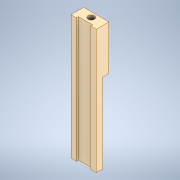
# Autodesk Inventor part: 5211_Bias_TxRx_Relative_Dovetail_Female_MPSv2_v4
Saved by Autodesk Inventor 2021 (Build 250183000, 183)
## iProperties
Created: 2020-11-13
Part Number: 5211_Bias_TxRx_Relative_Dovetail_Female_MPSv2_v4
Material: Polyethylene, High Density
Document SubType Name: Modeling
Designer: Admin
Density: 0.952 g/cm^3
Appearance: Smooth - Off-White
Author: Admin
Autodesk Inventor part; units mm, degrees
ref_plane "YZ Plane" through (0, 0, 0) normal (1, 0, 0) x (0, 1, 0)
ref_plane "XZ Plane" through (0, 0, 0) normal (0, 1, 0) x (-1, 0, 0)
ref_plane "XY Plane" through (0, 0, 0) normal (0, 0, 1) x (1, 0, 0)
sketch "Sketch1" plane through (0, 0, 0) normal (0, 0, 1) x (1, 0, 0)
  line L0 (0, 0) -> (47, 0)
  line L1 (47, 0) -> (47, -300)
  line L2 (47, -300) -> (0, -300)
  line L3 (0, -300) -> (0, 0)
  dimension "d0" = 47
  dimension "d1" = 300
  constraints: 8 end point, 2 parallel, 1 horizontal, 1 perpendicular
  measures "d0" distance of L1.end L2.end
  measures "d1" distance of L0.end L1.end
extrude "Extrusion1" add sketch "Sketch1" along normal blind 25.4
sketch "Sketch2" plane through (0, -300, 0) normal (0, -1, 0) x (1, 0, 0)
  line L0 (0, 0) -> (0, 25.4) projected
  line L1 (0, 25.4) -> (47, 25.4) projected
  line L2 (0, 0) -> (10, 0)
  line L3 (10, 0) -> (10, 21.4)
  line L4 (10, 25.4) -> (0, 25.4)
  line L5 (0, 25.4) -> (0, 0)
  line L6 (0, 0) -> (47, 0) projected
  line L7 (47, 0) -> (37, 0)
  line L8 (37, 0) -> (37, 25.4)
  line L9 (37, 25.4) -> (47, 25.4)
  line L10 (47, 25.4) -> (47, 0)
  line L11 (10, 25.4) -> (3.1941, 0)
  line L12 (10, 25.4) -> (36.296, 25.4) construction
  line L13 (37, 25.4) -> (43.8059, 0)
  line L14 (37, 25.4) -> (63.296, 25.4) construction
  line L15 (37, 25.4) -> (37, 21.4)
  line L16 (37, 21.4) -> (8.9282, 21.4)
  line L17 (37, 21.4) -> (38.0718, 21.4)
  line L18 (10, 25.4) -> (37, 25.4)
  dimension "d4" = 10
  dimension "d5" = 10
  dimension "d6" = 105
  dimension "d7" = 75
  dimension "d8" = 4
  constraints: 32 end point, 9 point on line, 5 horizontal, 4 parallel, 2 equal length, 2 perpendicular, 1 collinear
  measures "d4" distance of L4.end L4.start
  measures "d5" distance of L8.end L9.end
  measures "d6" angle of L11 L12
  measures "d7" angle of L13 L14
  measures "d8" distance of L8.end L15.end
extrude "Extrusion2" cut sketch "Sketch2" against normal blind 300 contours L1 L8 L16 L11 | L13 L17 L8
sketch "Sketch3" plane through (0, 0, 0) normal (0, 0, -1) x (-1, 0, 0)
  line L0 (-50.8, -30) -> (0, -30)
  line L1 (0, -30) -> (-50.8, -30)
  line L2 (0, 8.1) -> (0, -30)
  line L3 (-47, -30) -> (0, -30)
  line L4 (0, -15) -> (0, -30)
  line L5 (0, -30) -> (-47, -30)
  line L6 (-47, -30) -> (-47, -15)
  line L7 (-47, -15) -> (0, -15)
  line L8 (0, -15) -> (-47, -30) construction
  line L9 (0, -30) -> (-47, -15) construction
  line L10 (-47, 0) -> (0, 0)
  line L11 (0, 0) -> (-47, -15) construction
  line L12 (0, -15) -> (-47, 0) construction
  line L13 (-47, -15) -> (0, -15)
  line L14 (0, -15) -> (-47, -15)
  line L15 (0, 0) -> (0, -15)
  line L16 (-47, -15) -> (-47, 0)
  line L17 (-8.5, -22.5) -> (-8.5, -7.5)
  circle A0 centre (-8.5, -22.5) radius 1.5875
  circle A1 centre (-38.5, -22.5) radius 1.5875
  circle A2 centre (-38.5, -7.5) radius 1.5875
  circle A3 centre (-8.5, -7.5) radius 1.5875
  line L18 (-47, 0) -> (0, 0) projected
  line L19 (0, 0) -> (0, -122.988)
  line L20 (0, 0) -> (0, -300) projected
  line L21 (-50.8, -122.988) -> (0, -122.988)
  line L22 (0, -122.988) -> (-50.8, -122.988)
  line L23 (-47, -122.988) -> (0, -122.988)
  line L24 (0, -107.988) -> (0, -122.988)
  line L25 (0, -122.988) -> (-47, -122.988)
  line L26 (-47, -122.988) -> (-47, -107.988)
  line L27 (-47, -107.988) -> (0, -107.988)
  line L28 (0, -107.988) -> (-47, -122.988) construction
  line L29 (0, -122.988) -> (-47, -107.988) construction
  line L30 (-47, -92.988) -> (0, -92.988)
  line L31 (0, -92.988) -> (-47, -107.988) construction
  line L32 (0, -107.988) -> (-47, -92.988) construction
  line L33 (-47, -107.988) -> (0, -107.988)
  line L34 (0, -107.988) -> (-47, -107.988)
  line L35 (0, -92.988) -> (0, -107.988)
  line L36 (-47, -107.988) -> (-47, -92.988)
  line L37 (-8.5, -115.488) -> (-8.5, -100.488)
  circle A4 centre (-8.5, -115.488) radius 1.5875
  circle A5 centre (-38.5, -115.488) radius 1.5875
  circle A6 centre (-38.5, -100.488) radius 1.5875
  circle A7 centre (-8.5, -100.488) radius 1.5875
  line L38 (-16, -115.488) -> (-13.5, -115.488)
  line L39 (-13.5, -115.488) -> (-8.5, -115.488)
  line L40 (-31, -115.488) -> (-33.5, -115.488)
  line L41 (-33.5, -115.488) -> (-41, -115.488)
  line L42 (-41, -115.488) -> (-38.5, -115.488)
  point P0 (0, -6.35)
  point P1 (0, -30)
  point P2 (-27, -15)
  point P3 (-12, -15)
  point P4 (0, -15)
  point P5 (-10, 0)
  point P6 (0, -99.338)
  point P7 (-27, -107.988)
  point P8 (-12, -107.988)
  point P9 (0, -107.988)
  dimension "d11" = 15
  dimension "d12" = 15
  dimension "d13" = 3.175
  dimension "d14" = 3.175
  dimension "d15" = 3.175
  dimension "d16" = 3.175
  dimension "d17" = 122.988
  dimension "d18" = 15
  dimension "d19" = 15
  dimension "d20" = 3.175
  dimension "d21" = 3.175
  dimension "d22" = 3.175
  dimension "d23" = 3.175
  dimension "d30" = 5
  dimension "d31" = 7.5
  dimension "d32" = 2.5
  constraints: 82 end point, 8 centre point, 8 parallel, 4 coincident, 4 horizontal, 4 perpendicular, 3 point on line, 2 other
  measures "d11" distance of L3.start L6.end
  measures "d12" distance of L11.end L10.start
  measures "d13" diameter of A0
  measures "d14" diameter of A1
  measures "d15" diameter of A2
  measures "d16" diameter of A3
  measures "d17" distance of L18.end L19.end
  measures "d18" distance of L28.end L27.start
  measures "d19" distance of L33.start L32.end
  measures "d20" diameter of A4
  measures "d21" diameter of A5
  measures "d22" diameter of A6
  measures "d23" diameter of A7
  measures "d30" distance of L38.end L39.end
  measures "d31" distance of L40.end L41.end
  measures "d32" distance of L41.end L42.end
extrude "Extrusion3" cut sketch "Sketch3" against normal blind 10 contours A0 | A7 | A3 | A4 L39 L37 | L37 L39 A4 | A1 | A2 | L41 A5 | A5 L41 | A6
sketch "Sketch4" plane through (0, -300, 0) normal (0, -1, 0) x (1, 0, 0)
  line L0 (0, 0) -> (47, 0) projected
  line L1 (47, 0) -> (47, 25.4) projected
  line L2 (0, 0) -> (47, 0)
  line L3 (47, 0) -> (47, 12.7)
  line L4 (47, 12.7) -> (0, 12.7)
  line L5 (0, 12.7) -> (0, 0)
  dimension "d27" = 12.7
  constraints: 8 end point, 2 parallel, 1 horizontal, 1 midpoint, 1 perpendicular
  measures "d27" distance of L3.end L2.end
extrude "Extrusion4" cut sketch "Sketch4" against normal blind 160
sketch "Sketch7" plane through (0, 0, 0) normal (0, 1, 0) x (1, 0, 0)
  line L0 (47, -25.4) -> (37, -25.4) projected
  line L1 (0, 0) -> (47, -25.4)
  line L2 (47, -25.4) -> (47, 0)
  line L3 (10, -25.4) -> (0, -25.4) projected
  line L4 (47, 0) -> (0, -25.4)
  circle A0 centre (23.5, -12.7) radius 6.35
  line L5 (23.5, -12.7) -> (21, -12.7)
  line L6 (0, -12.7) -> (47, -12.7) projected
  line L7 (23.5, -12.7) -> (23.5, -10.2)
  line L8 (23.5, -12.7) -> (26, -12.7) construction
  circle A1 centre (23.5, -10.2) radius 6.35
  dimension "d33" = 12.7
  dimension "d34" = 2.5
  dimension "d35" = 2.5
  dimension "d36" = 90
  dimension "d37" = 12.7
  constraints: 12 end point, 3 perpendicular, 2 centre point, 1 coincident, 1 horizontal, 1 midpoint, 1 point on line
  measures "d33" diameter of A0
  measures "d34" distance of L5.start L5.end
  measures "d35" distance of L5.start L7.end
  measures "d36" angle of L8 L7
  measures "d37" diameter of A1
extrude "Extrusion5" cut sketch "Sketch7" against normal blind 100 contours A1 L4 A0 L1 | L1 A0 A1 | A0 L4 L1 | L1 L5 L6 A1 A0 | A1 A0 L4 | L6 A1 L1 | L1 A1 L4 | L4 A1 L6 L5 | L4 A0 A1 L6 picked at (23.5, -5.5468) picked at (27.3983, -11.8828)
sketch "Sketch9" plane through (0, 0, 0) normal (0, 0, -1) x (-1, 0, 0)
  circle A0 centre (-38.5, -22.5) radius 1.5875 projected
  circle A1 centre (-38.5, -100.488) radius 1.5875 projected
  line L0 (-38.5, -22.5) -> (-38.5, -100.488)
  line L1 (-38.5, -100.488) -> (-38.5, -62.7)
  circle A2 centre (-38.5, -115.488) radius 1.5875 projected
  line L2 (-38.5, -115.488) -> (-38.5, -77.7)
  circle A3 centre (-38.5, -62.7) radius 1.5875
  circle A4 centre (-38.5, -77.7) radius 1.5875
  line L3 (-38.5, -100.488) -> (-8.5476, -100.488)
  line L4 (-38.5, -77.7) -> (-8.4125, -77.7)
  circle A5 centre (-8.4125, -62.7) radius 1.5875
  circle A6 centre (-8.4125, -77.7) radius 1.5875
  line L5 (-10, -62.7) -> (-11.5875, -62.7)
  point P0 (0, 0)
  dimension "d40" = 37.788
  dimension "d41" = 37.788
  dimension "d42" = 3.175
  dimension "d43" = 3.175
  dimension "d44" = 3.175
  dimension "d45" = 3.175
  dimension "d59" = 1.5875
  constraints: 12 end point, 4 centre point, 3 coincident, 2 point on line, 1 horizontal, 1 vertical
  measures "d40" distance of L0.end L1.end
  measures "d41" distance of L2.start L2.end
  measures "d42" diameter of A3
  measures "d43" diameter of A4
  measures "d44" diameter of A5
  measures "d45" diameter of A6
  measures "d59" distance of L5.start L5.end
extrude "Extrusion6" cut sketch "Sketch9" against normal blind 10 contours A6 | A4 L4 L0 | L0 A4 | A3 L0 | L0 A3 | L4 A4 L0 | A5
sketch "Sketch10" plane through (0, 0, 0) normal (0, 0, -1) x (-1, 0, 0)
  line L0 (-47, -140) -> (-47, 0) projected
  line L1 (0, 0) -> (-47, 0)
  line L2 (-47, 0) -> (-47, -50)
  line L3 (-47, -50) -> (0, -50)
  line L4 (0, -50) -> (0, 0)
  point P0 (-47, 0)
  dimension "d48" = 50
  constraints: 8 end point, 2 parallel, 1 horizontal, 1 perpendicular, 1 point on line
  measures "d48" distance of L2.end L1.end
extrude "Extrusion7" cut sketch "Sketch10" against normal blind 30
sketch "Sketch11" plane through (0, 0, 0) normal (0, 0, -1) x (-1, 0, 0)
  line L0 (-10, -50) -> (0, -50) projected
  line L1 (0, -50) -> (1.9, -50)
  line L2 (0, -50) -> (-47, -50) projected
  line L3 (-47, -50) -> (-48.9, -50)
  line L4 (-48.9, -50) -> (-48.9, -300)
  line L5 (-37, -300) -> (-47, -300) projected
  line L6 (-47, -300) -> (-48.9, -300)
  line L7 (-47, -300) -> (-47, -50) projected
  line L8 (-47, -50) -> (-47, -300)
  line L9 (0, -50) -> (0, -300) projected
  line L10 (0, -50) -> (0, -300)
  line L11 (0, -300) -> (0, -298.1)
  line L12 (1.9, -300) -> (0, -300)
  line L13 (1.9, -300) -> (1.9, -50)
  point P0 (0, 0)
  dimension "d51" = 1.9
  dimension "d52" = 1.9
  dimension "d53" = 1.9
  constraints: 18 end point, 3 horizontal, 3 perpendicular, 2 collinear, 1 point on line
  measures "d51" distance of L0.end L1.end
  measures "d52" distance of L2.end L3.end
  measures "d53" distance of L9.end L11.end
extrude "Extrusion8" add sketch "Sketch11" against normal blind 25.4
sketch "Sketch12" plane through (0, 0, 0) normal (0, 0, -1) x (-1, 0, 0)
  line L0 (-37, -300) -> (-48.9, -300) projected
  line L1 (1.9, -50) -> (1.9, -300) projected
  line L2 (-48.9, -300) -> (1.9, -300)
  line L3 (1.9, -300) -> (1.9, -140)
  line L4 (1.9, -140) -> (-48.9, -140)
  line L5 (-48.9, -140) -> (-48.9, -300)
  point P0 (0, 0)
  dimension "d56" = 160
  constraints: 8 end point, 2 parallel, 1 horizontal, 1 perpendicular, 1 point on line
  measures "d56" distance of L3.end L2.end
extrude "Extrusion9" cut sketch "Sketch12" against normal blind 12.7
body "Solid1"
